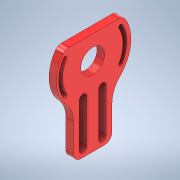
# Autodesk Inventor part: part12
Saved by Autodesk Inventor 2021 (Build 250183000, 183)
## iProperties
Created: 2022-04-30
Part Number: part12
Material: Generic
Document SubType Name: Modeling
Designer: authe
Density: 1 g/cm^3
Appearance: Light Red
Author: authe
Autodesk Inventor part; units mm, degrees
ref_plane "YZ Plane" through (0, 0, 0) normal (1, 0, 0) x (0, 1, 0)
ref_plane "XZ Plane" through (0, 0, 0) normal (0, 1, 0) x (-1, 0, 0)
ref_plane "XY Plane" through (0, 0, 0) normal (0, 0, 1) x (1, 0, 0)
sketch "Sketch1" plane through (0, 0, 0) normal (1, 0, 0) x (0, 1, 0)
  point P0 (0, 0)
sketch "Sketch2" plane through (0, 0, 0) normal (1, 0, 0) x (0, 1, 0)
  circle A0 centre (0, 0) radius 31.5
  arc A1 (40, 69.282) -> (-40, 69.282) centre (0, 0) ccw
  line L0 (0, 0) -> (-40, 69.282) construction
  line L1 (0, 0) -> (80, 0) construction
  line L2 (0, 0) -> (40, 69.282) construction
  line L3 (40, 69.282) -> (45, 77.9423)
  line L4 (-40, 69.282) -> (-45, 77.9423)
  arc A2 (40, 69.282) -> (45, 77.9423) centre (42.5, 73.6122) ccw
  arc A3 (-45, 77.9423) -> (-40, 69.282) centre (-42.5, 73.6122) ccw
  arc A4 (-40, -69.282) -> (40, -69.282) centre (0, 0) ccw
  line L5 (0, 0) -> (40, -69.282) construction
  line L6 (0, 0) -> (80, 0) construction
  line L7 (0, 0) -> (-40, -69.282) construction
  line L8 (-40, -69.282) -> (-45, -77.9423)
  arc A5 (45, -77.9423) -> (40, -69.282) centre (42.5, -73.6122) ccw
  arc A6 (-40, -69.282) -> (-45, -77.9423) centre (-42.5, -73.6122) ccw
  arc A7 (45, 77.9423) -> (-45, 77.9423) centre (0, 0) ccw
  arc A8 (-45, -77.9423) -> (45, -77.9423) centre (0, 0) ccw
  arc A9 (40, 69.282) -> (-40, 69.282) centre (0, 0) ccw
  arc A10 (-40, -69.282) -> (40, -69.282) centre (0, 0) ccw
  line L9 (0, 0) -> (-72.5, 0)
  line L10 (-72.5, 0) -> (-72.5, -15.5)
  line L11 (-72.5, -15.5) -> (-72.5, -35.5)
  line L12 (-72.5, -35.5) -> (-72.5, -51)
  line L13 (-121.003, -51) -> (-188, -51)
  line L14 (-188, -51) -> (-188, -35.5)
  line L15 (-188, -35.5) -> (-72.5, -35.5)
  line L16 (-72.5, -15.5) -> (-188, -15.5)
  line L17 (-188, -15.5) -> (-188, -35.5)
  circle A11 centre (-72.5, -25.5) radius 10
  circle A12 centre (-188, -25.5) radius 10
  line L18 (-72.5, 0) -> (-72.5, 15.5)
  line L19 (-72.5, 15.5) -> (-72.5, 35.5)
  line L20 (-72.5, 35.5) -> (-72.5, 51)
  line L21 (-112.428, 51) -> (-188, 51)
  line L22 (-188, 51) -> (-188, 35.5)
  line L23 (-188, 35.5) -> (-72.5, 35.5)
  line L24 (-72.5, 15.5) -> (-188, 15.5)
  line L25 (-188, 15.5) -> (-188, 35.5)
  circle A13 centre (-188, 25.5) radius 10
  circle A14 centre (-72.5, 25.5) radius 10
  line L26 (-188, 51) -> (-188, 51)
  line L27 (-208, 31) -> (-208, -31)
  line L28 (-188, -51) -> (-188, -51)
  arc A15 (-208, -31) -> (-188, -51) centre (-188, -31) ccw
  arc A16 (-188, 51) -> (-208, 31) centre (-188, 31) ccw
  line L29 (-188, 25.5) -> (-72.5, 25.5)
  arc A17 (-98.8167, 35.5) -> (-103.8497, 15.5) centre (0, 0) ccw
  arc A18 (-71.5049, -71.5031) -> (-121.003, -51) centre (-121.003, -121) ccw
  arc A19 (-112.428, 51) -> (-68.365, 66.6083) centre (-112.428, 121) ccw
  line L30 (0, 0) -> (62.5, 0)
  line L31 (62.5, 0) -> (62.5, 62.3398)
  line L32 (62.5, 0) -> (62.5, -69.098)
  arc A20 (-71.5049, -71.5031) -> (52.978, -86.1335) centre (0, 0) ccw
  arc A21 (53.7659, 78.8649) -> (-68.365, 66.6083) centre (0, 0) ccw
  arc A22 (62.5, 62.3398) -> (53.7659, 78.8649) centre (42.5, 62.3398) ccw
  arc A23 (52.978, -86.1335) -> (62.5, -69.098) centre (42.5, -69.098) ccw
  point P0 (-208, 51)
  point P1 (-87.3193, 51)
  point P2 (-87.3193, -51)
  point P3 (62.5, 72.1401)
  point P4 (62.5, -79.4947)
  dimension "d0" = 63
  dimension "d4" = 120
  dimension "d5" = 60
  dimension "d6" = 60
  dimension "d7" = 60
  dimension "d8" = 10
  dimension "d9" = 10
  dimension "d10" = 72.5
  dimension "d11" = 15.5
  dimension "d12" = 20
  dimension "d13" = 15.5
  dimension "d14" = 115.5
  dimension "d15" = 15.5
  dimension "d16" = 20
  dimension "d17" = 15.5
  dimension "d18" = 20
  dimension "d20" = 20
  dimension "d21" = 20
  dimension "d22" = 115.5
  dimension "d23" = 70
  dimension "d24" = 70
  dimension "d25" = 62.5
  dimension "d26" = 20
  dimension "d27" = 20
  constraints: 66 end point, 42 point on circle, 21 centre point, 18 point on line, 12 perpendicular, 11 tangent, 7 midpoint, 6 coincident, 5 horizontal, 2 equal length, 2 parallel, 1 vertical, 9 other
  measures "d0" diameter of A0
  measures "d4" angle of L1 L0
  measures "d5" angle of L2 L0
  measures "d6" angle of L5 L6
  measures "d7" angle of L7 L5
  measures "d8" diameter of A5
  measures "d9" diameter of A6
  measures "d10" distance of L5.start L9.end
  measures "d11" distance of L9.end L10.end
  measures "d12" distance of L10.end L11.end
  measures "d13" distance of L11.end L12.end
  measures "d14" distance of L12.end L13.end
  measures "d15" distance of L9.end L18.end
  measures "d16" distance of L18.end L19.end
  measures "d17" distance of L19.end L20.end
  measures "d18" distance of L21.end point (-208, 51)
  measures "d20" radius of A15
  measures "d21" radius of A16
  measures "d22" distance of L29.start L29.end
  measures "d23" radius of A18
  measures "d24" radius of A19
  measures "d25" distance of L5.start L30.end
  measures "d26" radius of A22
  measures "d27" radius of A23
extrude "Extrusion1" add sketch "Sketch2" along normal blind 20 contours L30 L32 A23 A20 A18 L13 L14 L15 A11 L10 L9 A0 | A0 L9 L18 A14 L23 L22 L21 A19 A21 A22 L31 L30 | L10 L16 A12 L14 A15 L27 A16 L22 A13 L24 L18
body "Solid1"
